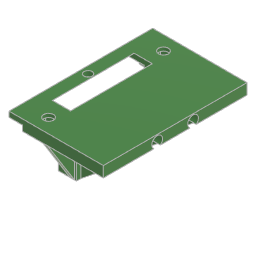
plate_bracket v2 (Autodesk Fusion 360 design; units mm, degrees)
Autodesk Fusion 360 part; units mm, degrees
note: some values were not read from the file. Chosen so that the rebuilt part matches the saved one: a direction; which face or edge a step refers to. Set by a fixed rule: which sketch regions a step uses.
sketch "Sketch1" plane through (0, 0, 0) normal (1, 0, 0) x (0, 1, 0)
  line L0 (0, 0) -> (50, 0)
  line L1 (50, 0) -> (50, 30)
  line L2 (50, 30) -> (0, 30)
  line L3 (0, 30) -> (0, 0)
  dimension "d1" = 50
  dimension "d2" = 30
  constraint horizontal L0
  constraint vertical L1
  constraint horizontal L2
  constraint vertical L3
  constraint coincident L0.start L3.end
  measures "d1" distance of L0.start L0.end
  measures "d2" distance of L0.start L2.end
extrude "Extrude1" add sketch "Sketch1" along normal blind 10
sketch "Sketch2" plane through (0, 0, 0) normal (-1, 0, 0) x (0, -1, 0)
  line L0 (0, 0) -> (0, 30)
  line L1 (0, 30) -> (-50, 30)
  line L2 (-50, 30) -> (-50, 0)
  line L3 (-50, 0) -> (0, 0)
  line L4 (-25, 30) -> (-25, 0) construction
  line L5 (-47.75, 30) -> (-2.25, 30)
  line L6 (-2.25, 30) -> (-2.25, 2.9)
  line L7 (-2.25, 2.9) -> (-47.75, 2.9)
  line L8 (-47.75, 2.9) -> (-47.75, 30)
  line L9 (-25, 30) -> (-25, 2.9) construction
  line L10 (-15, 6.45) -> (-35, 6.45) construction
  line L11 (-35, 6.45) -> (-35, 26.45) construction
  line L12 (-35, 26.45) -> (-15, 26.45) construction
  line L13 (-15, 26.45) -> (-15, 6.45) construction
  line L14 (-15, 6.45) -> (-35, 26.45) construction
  line L15 (-35, 6.45) -> (-15, 26.45) construction
  point P0 (-25, 16.45)
  dimension "d5" = 27.1
  dimension "d6" = 45.5
  dimension "d7" = 20
  dimension "d8" = 20
  constraint midpoint L1 L4.start
  constraint midpoint L3 L4.end
  constraint horizontal L5
  constraint vertical L6
  constraint horizontal L7
  constraint vertical L8
  constraint coincident L1 L5.start
  constraint midpoint L5 L4.start
  constraint midpoint L7 L9.end
  constraint collinear L4 L9
  constraint horizontal L10
  constraint perpendicular L10 L11
  constraint parallel L10 L12
  constraint parallel L11 L13
  constraint coincident L14 P0
  constraint coincident L15 P0
  constraint midpoint L9 P0
  measures "d5" distance of L5.start L7.end
  measures "d6" distance of L6 L8
  measures "d7" distance of L11.end L12.end
  measures "d8" distance of L10.end L11.end
extrude "Extrude2" cut sketch "Sketch2" against normal blind 4.5 contours L1 L5 L6 L7 L8
hole "Hole1" at (0, 35, 26.45) at (0, 15, 6.45) at (0, 35, 6.45) at (0, 15, 26.45) direction (1, 0, 0) diameter 3.4 end through all
sketch "Sketch3" plane through (0, 0, 30) normal (0, 0, 1) x (-1, 0, 0)
  line L0 (0, -47.75) -> (-4.5, -47.75)
  line L1 (-4.5, -47.75) -> (-4.5, -2.25)
  line L2 (-4.5, -2.25) -> (0, -2.25)
  line L3 (0, -2.25) -> (0, 0)
  line L4 (0, 0) -> (-10, 0)
  line L5 (-10, 0) -> (-10, -50)
  line L6 (-10, -50) -> (0, -50)
  line L7 (0, -50) -> (0, -47.75)
  line L8 (-4.5, -47.75) -> (-4.5, -2.25)
  line L9 (-4.5, -2.25) -> (5.6, -2.25)
  line L10 (5.6, -2.25) -> (5.6, -47.75)
  line L11 (5.6, -47.75) -> (-4.5, -47.75)
  line L12 (-10, -25) -> (49, -25) construction
  line L13 (-10, -65) -> (12.5, -65)
  line L14 (12.5, -65) -> (12.5, 15)
  line L15 (12.5, 15) -> (-10, 15)
  line L16 (-10, 15) -> (-10, -65)
  line L17 (12.5, -25) -> (-10, -25) construction
  dimension "d14" = 10.1
  dimension "d15" = 22.5
  constraint perpendicular L8 L9
  constraint parallel L8 L10
  constraint parallel L9 L11
  constraint coincident L1.end L2.start
  constraint perpendicular L2 L8
  constraint coincident L0.end L1.start
  constraint midpoint L5 L12.start
  constraint perpendicular L5 L12
  constraint horizontal L13
  constraint vertical L14
  constraint horizontal L15
  constraint vertical L16
  constraint midpoint L14 L17.start
  constraint midpoint L16 L12.start
  constraint collinear L12 L17
  measures "d14" distance of L0.end L10.end
  measures "d15" distance of L13.start L13.end
extrude "Extrude3" add sketch "Sketch3" against normal blind 3 contours L3 L4 L6 L7 L9 L10 L11 L13 L14 L15 L16
sketch "Sketch4" plane through (0, 0, 27) normal (0, 0, -1) x (1, 0, 0)
  line L0 (10, -65) -> (10, -50)
  line L1 (10, -50) -> (0, -50)
  line L2 (0, -50) -> (0, -47.75)
  line L3 (0, -47.75) -> (-5.6, -47.75)
  line L4 (-5.6, -47.75) -> (-5.6, -2.25)
  line L5 (-5.6, -2.25) -> (0, -2.25)
  line L6 (0, -2.25) -> (0, 0)
  line L7 (0, 0) -> (10, 0)
  line L8 (10, 0) -> (10, 15)
  line L9 (10, 15) -> (-12.5, 15)
  line L10 (-12.5, 15) -> (-12.5, -65)
  line L11 (-12.5, -65) -> (10, -65)
  line L12 (10, 0) -> (-5, 0)
  line L13 (-5, 0) -> (-5, 15)
  line L14 (-5, 15) -> (10, 15)
  line L15 (10, 15) -> (10, 0)
  line L16 (10, -65) -> (-5, -65)
  line L17 (-5, -65) -> (-5, -50)
  line L18 (-5, -50) -> (10, -50)
  line L19 (10, -50) -> (10, -65)
  dimension "d31" = 15
  constraint horizontal L12
  constraint vertical L13
  constraint horizontal L14
  constraint vertical L15
  constraint coincident L9 L13.end
  constraint coincident L7.end L8.start
  constraint horizontal L16
  constraint vertical L17
  constraint horizontal L18
  constraint vertical L19
  constraint coincident L0.start L11.end
  measures "d31" distance of L13 L15
extrude "Extrude4" add sketch "Sketch4" along normal blind 3 contours L0 L1 L11 L16 L17 L18 L19 | L7 L8 L9 L12 L13 L14 L15
sketch "Sketch5" plane through (0, 0, 24) normal (0, 0, -1) x (1, 0, 0)
  line L0 (10, 15) -> (-5, 15)
  line L1 (-5, 15) -> (-5, 0)
  line L2 (0, 0) -> (10, 0)
  line L3 (10, 0) -> (10, 15)
  line L4 (1.5, 15) -> (1.5, -65) construction
  line L5 (5.425, 9.2661) -> (1.5, 11.5322)
  line L6 (1.5, 11.5322) -> (-2.425, 9.2661)
  line L7 (-2.425, 9.2661) -> (-2.425, 4.7339)
  line L8 (-2.425, 4.7339) -> (1.5, 2.4678)
  line L9 (1.5, 2.4678) -> (5.425, 4.7339)
  line L10 (5.425, 4.7339) -> (5.425, 9.2661)
  line L11 (5.425, -54.7339) -> (1.5, -52.4678)
  line L12 (1.5, -52.4678) -> (-2.425, -54.7339)
  line L13 (-2.425, -54.7339) -> (-2.425, -59.2661)
  line L14 (-2.425, -59.2661) -> (1.5, -61.5322)
  line L15 (1.5, -61.5322) -> (5.425, -59.2661)
  line L16 (5.425, -59.2661) -> (5.425, -54.7339)
  line L17 (-5, 0) -> (0, 0)
  point P0 (1.5, 7)
  point P1 (1.5, -57)
  point P2 (-8.5, -25)
  dimension "d21" = 8.5
  dimension "d22" = 3.925
  dimension "d23" = 3.925
  dimension "d24" = 64
  dimension "d25" = 8
  dimension "d32" = 32
  dimension "d33" = 10
  constraint coincident L0 L4.start
  constraint perpendicular L0 L4
  constraint coincident L4 P0
  constraint vertical L10
  constraint coincident L4 P1
  constraint vertical L16
  measures "d21" distance of L3 L4
  measures "d22" distance of P0 L10
  measures "d23" distance of P1 L16
  measures "d24" distance of P0 P1
  measures "d25" distance of L0 P0
  measures "d32" vertical distance of P0 P2
  measures "d33" horizontal distance of P0 P2
hole "Hole2" at (1.5, -7, 24) at (1.5, 57, 24) direction (0, 0, 1) diameter 5.5 depth 10 tip angle 118
extrude "Extrude5" cut sketch "Sketch5" against normal blind 4 contours L5 L6 L7 L8 L9 L10 | L11 L12 L13 L14 L15 L16
hole "Hole3" at (-8.5, 25, 24) direction (0, 0, 1) diameter 4.5 depth 10 tip angle 118
ref_plane "WorkPlane1" through (7.7125, -7, 26) normal (-1, 0, 0) x (0, -1, 0)
sketch "Sketch6" plane through (7.7125, -7, 26) normal (-1, 0, 0) x (0, 1, 0)
  line L0 (-8, 2) -> (7, 26)
  line L1 (57, 26) -> (72, 2)
rib "Rib1" add thickness 2.5 on both sides direction (0, 0.847998, 0.529999) up to next extending the curves path "Sketch6" along L0
rib "Rib2" add thickness 2.5 on both sides direction (0, -0.847998, 0.529999) up to next extending the curves path "Sketch6" along L1
chamfer "Chamfer1" distance 3 angle 45 1 edges at (-5.6, 25, 27)
chamfer "Chamfer2" distance 2.9 distance2 4.5 1 edges at (0, 25, 2.9) measured on face at (0, 17.4167, 0.9667)
sketch "Sketch7" plane through (10, 0, 0) normal (1, 0, 0) x (0, 1, 0)
  circle A0 centre (35, 6.45) radius 1.7
  circle A1 centre (35, 26.45) radius 1.7
  circle A2 centre (15, 6.45) radius 1.7
  circle A3 centre (15, 26.45) radius 1.7
  line L0 (0, 24) -> (0, 0)
  line L1 (0, 0) -> (50, 0)
  line L2 (50, 0) -> (50, 24)
  line L3 (50, 24) -> (65, 24)
  line L4 (65, 24) -> (65, 30)
  line L5 (65, 30) -> (-15, 30)
  line L6 (-15, 30) -> (-15, 24)
  line L7 (-15, 24) -> (0, 24)
  line L8 (25, 0) -> (25, 30) construction
  line L9 (-15, 30) -> (65, 30)
  line L10 (65, 30) -> (65, 24)
  line L11 (65, 24) -> (-15, 24)
  line L12 (-15, 24) -> (-15, 30)
  circle A4 centre (15, 26.45) radius 3
  circle A5 centre (35, 26.45) radius 3
  dimension "d45" = 6
  dimension "d46" = 6
  constraint midpoint L1 L8.start
  constraint midpoint L5 L8.end
  constraint horizontal L9
  constraint vertical L10
  constraint horizontal L11
  constraint vertical L12
  constraint coincident L5.end L6.start
  constraint collinear L4 L10
  constraint concentric A3 A4
  constraint concentric A1 A5
  measures "d45" diameter of A5
  measures "d46" diameter of A4
extrude "Extrude6" add sketch "Sketch7" along normal blind 30 contours L3 L4 L5 L6 L7 L9 L10 L11 L12 A4 A5
ref_plane "WorkPlane2" through (13.75, 5, 27) normal (0, -1, 0) x (-1, 0, 0)
ref_plane "WorkPlane3" through (13.75, 45, 27) normal (0, 1, 0) x (1, 0, 0)
ref_plane "WorkPlane4" through (13.75, 25, 27) normal (0, 1, 0) x (1, 0, 0)
sketch "Sketch8" plane through (10, 5, 27) normal (0, -1, 0) x (1, 0, 0)
  line L0 (0, -27) -> (30, -3)
sketch "Sketch9" plane through (10, 25, 27) normal (0, 1, 0) x (1, 0, 0)
  line L0 (0, 27) -> (30, 3)
sketch "Sketch10" plane through (10, 45, 27) normal (0, 1, 0) x (1, 0, 0)
  line L0 (0, 27) -> (30, 3)
rib "Rib3" add thickness 5 on both sides direction (-0.624695, 0, 0.780869) up to next extending the curves path "Sketch8" along L0
rib "Rib4" add thickness 5 on both sides direction (-0.624695, 0, 0.780869) up to next extending the curves path "Sketch9" along L0
rib "Rib5" add thickness 5 on both sides direction (-0.624695, 0, 0.780869) up to next extending the curves path "Sketch10" along L0
equation "d22 = ( 7.85 / 2 ) * 1 mm"
equation "d25 = ( ( 80 - 64 ) / 2 ) * 1 mm"
